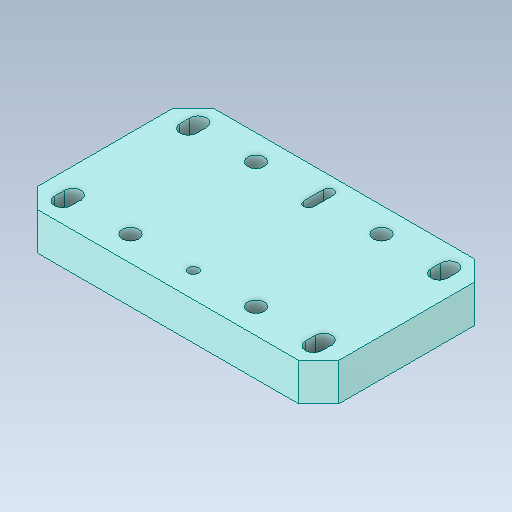
# Autodesk Inventor part: FAB-P0001
Saved by Autodesk Inventor 2020 (Build 240168000, 168)
## iProperties
Created: 2012-05-14
Part Number: FAB-P0001
Material: SolidWorks Materials|6061-T6 (SS)
Description: Stage vertical support base
Document SubType Name: Modeling
Designer: map
Density: 2.7 g/cm^3
Appearance: 192,255,255
Company: RESOLUTION DEVELOPMENT SERVICES
Sending System: SolidWorks 2015
Last Author: yl862
Last Saved: 2016-06-16
Author: map
Revision Number: 02
Title: Stage vertical support base
Autodesk Inventor part; units mm, degrees
ref_plane "YZ Plane" through (0, 0, 0) normal (1, 0, 0) x (0, 1, 0)
ref_plane "XZ Plane" through (0, 0, 0) normal (0, 1, 0) x (-1, 0, 0)
ref_plane "XY Plane" through (0, 0, 0) normal (0, 0, 1) x (1, 0, 0)
sketch "Sketch1" plane through (-52, 0, -35) normal (0, -1, 0) x (1, 0, 0)
  line L0 (0, 70) -> (104, 70) projected
  line L1 (104, 70) -> (112, 62) projected
  line L2 (112, 62) -> (112, 8) projected
  line L3 (112, 8) -> (104, 0) projected
  line L4 (104, 0) -> (0, 0) projected
  line L5 (0, 0) -> (-8, 8) projected
  line L6 (-8, 8) -> (-8, 62) projected
  line L7 (-8, 62) -> (0, 70) projected
  circle A0 centre (27, 10) radius 5.5 projected
  circle A1 centre (27, 60) radius 5.5 projected
  circle A2 centre (77, 60) radius 5.5 projected
  circle A3 centre (77, 10) radius 5.5 projected
  circle A4 centre (52, 60) radius 2 projected
  arc A5 (50, 6) -> (54, 6) centre (52, 6) ccw projected
  line L8 (54, 6) -> (54, 14) projected
  arc A6 (54, 14) -> (50, 14) centre (52, 14) ccw projected
  line L9 (50, 14) -> (50, 6) projected
  circle A7 centre (77, 35) radius 2 projected
  arc A8 (23, 37) -> (23, 33) centre (23, 35) ccw projected
  line L10 (23, 33) -> (31, 33) projected
  arc A9 (31, 33) -> (31, 37) centre (31, 35) ccw projected
  line L11 (31, 37) -> (23, 37) projected
  arc A10 (66.5, 62.5) -> (62.5, 62.5) centre (64.5, 62.5) ccw projected
  line L12 (62.5, 62.5) -> (62.5, 7.5) projected
  arc A11 (62.5, 7.5) -> (66.5, 7.5) centre (64.5, 7.5) ccw projected
  line L13 (66.5, 7.5) -> (66.5, 62.5) projected
  arc A12 (105.3, 62) -> (98.7, 62) centre (102, 62) ccw projected
  line L14 (98.7, 62) -> (98.7, 58) projected
  arc A13 (98.7, 58) -> (105.3, 58) centre (102, 58) ccw projected
  line L15 (105.3, 58) -> (105.3, 62) projected
  arc A14 (5.3, 62) -> (-1.3, 62) centre (2, 62) ccw projected
  line L16 (-1.3, 62) -> (-1.3, 58) projected
  arc A15 (-1.3, 58) -> (5.3, 58) centre (2, 58) ccw projected
  line L17 (5.3, 58) -> (5.3, 62) projected
  arc A16 (-1.3, 8) -> (5.3, 8) centre (2, 8) ccw projected
  line L18 (5.3, 8) -> (5.3, 12) projected
  arc A17 (5.3, 12) -> (-1.3, 12) centre (2, 12) ccw projected
  line L19 (-1.3, 12) -> (-1.3, 8) projected
  arc A18 (98.7, 8) -> (105.3, 8) centre (102, 8) ccw projected
  line L20 (105.3, 8) -> (105.3, 12) projected
  arc A19 (105.3, 12) -> (98.7, 12) centre (102, 12) ccw projected
  line L21 (98.7, 12) -> (98.7, 8) projected
  point P0 (52, 35)
extrude "Extrusion1" add sketch "Sketch1" against normal up to surface (15 mm away) contours L0 L1 L2 L3 L4 L5 L6 L7 | A0 | A1 | A2 | A3 | A4 | L9 A6 L8 A5 | A7 | L11 A9 L10 A8 | L13 A11 L12 A10 | L15 A13 L14 A12 | L17 A15 L16 A14 | L19 A17 L18 A16 | L21 A19 L20 A18
hole "M6CBore" at (25, 0, -25) at (-25, 0, -25) at (-25, 0, 25) at (25, 0, 25) direction (0, 1, 0) diameter 6.6 end through all counterbore diameter 11 counterbore depth 6.8 clearance for "Socket Head Cap Screw ISO 4762" size "M6" standard "ISO"
extrude "M6ClearanceSlots" cut sketch "Sketch1" against normal through all contours L15 A13 L14 A12 | L17 A15 L16 A14 | L19 A17 L18 A16 | L21 A19 L20 A18
sketch "Sketch2" plane through (-52, 15, -35) normal (0, 1, 0) x (1, 0, 0)
  line L0 (52, -14) -> (52, -6) construction
  line L1 (54, -14) -> (54, -6)
  line L2 (50, -6) -> (50, -14)
  arc A0 (50, -14) -> (54, -14) centre (52, -14) ccw
  arc A1 (54, -6) -> (50, -6) centre (52, -6) ccw
  point P0 (52, -35)
  point P1 (52, -60)
  point P2 (52, -10)
  dimension "d11" = 4
  constraints: 8 end point, 4 point on circle, 4 tangent, 2 centre point, 1 midpoint, 1 parallel, 1 vertical
  measures "d11" diameter of A1
hole "Hole2" at (0, 15, 25) direction (0, -1, 0) diameter 4 depth 8 tip angle 118
extrude "Extrusion3" cut sketch "Sketch2" against normal blind 8
body "Solid1"
